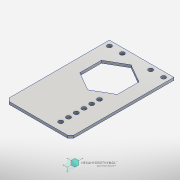
# Autodesk Inventor part: Z-head-topplate
Saved by Autodesk Inventor 2016 (Build 200138000, 138)
## iProperties
Created: 2015-05-16
Part Number: Z-head-topplate
Material: Aluminum 6061
Document SubType Name: Modeling
Designer: as
Mass: 17.1163 g
Surface Area: 72.6872 cm^2
Volume: 6.33935 cm^3
Density: 2.7 g/cm^3
Appearance: Aluminum - Flat
Author: as
Autodesk Inventor part; units mm, degrees
ref_plane "YZ Plane" through (0, 0, 0) normal (1, 0, 0) x (0, 1, 0)
ref_plane "XZ Plane" through (0, 0, 0) normal (0, 1, 0) x (-1, 0, 0)
ref_plane "XY Plane" through (0, 0, 0) normal (0, 0, 1) x (1, 0, 0)
sketch "Sketch1" plane through (0, 0, 0) normal (0, 0, 1) x (1, 0, 0)
  line L0 (0, 0) -> (50, 0)
  line L1 (50, 0) -> (50, -80)
  line L2 (50, -80) -> (0, -80)
  line L3 (0, -80) -> (0, 0)
  dimension "d0" = 50
  dimension "d1" = 80
  constraints: 8 end point, 2 parallel, 1 horizontal, 1 perpendicular
  measures "d0" distance of L1.end L2.end
  measures "d1" distance of L0.end L1.end
extrude "Extrusion1" add sketch "Sketch1" along normal blind 2
sketch "Sketch2" plane through (0, 0, 2) normal (0, 0, 1) x (1, 0, 0)
  point P0 (36, -4)
  point P1 (14, -4)
  point P2 (4, -4)
  point P3 (46, -4)
hole "Hole1" at (36, -4, 2) at (14, -4, 2) at (4, -4, 2) at (46, -4, 2) direction (0, 0, -1) diameter 3.4 depth 2
sketch "Sketch3" plane through (0, 0, 2) normal (0, 0, 1) x (1, 0, 0)
  point P0 (36, -43.66)
hole "Hole3" at (36, -43.66, 2) direction (0, 0, -1) diameter 3.4 depth 2
sketch "Sketch4" plane through (0, 0, 2) normal (0, 0, 1) x (1, 0, 0)
  line L0 (39.5492, -16.6) -> (39.5492, -33.4)
  line L1 (39.5492, -33.4) -> (25, -41.8)
  line L2 (25, -41.8) -> (10.4508, -33.4)
  line L3 (10.4508, -33.4) -> (10.4508, -16.6)
  line L4 (10.4508, -16.6) -> (25, -8.2)
  line L5 (25, -8.2) -> (39.5492, -16.6)
  line L6 (50, -80) -> (50, 0) projected
  line L7 (0, -80) -> (50, -80) projected
  line L8 (50, 0) -> (0, 0) construction
  line L9 (0, 0) -> (0, -80) construction
  point P0 (25, -25)
  dimension "d20" = 16.8
  dimension "d24" = 25
  dimension "d25" = 55
  dimension "d27" = 25
  dimension "d30" = 8.2
  constraints: 12 end point, 1 parallel, 13 other
  measures "d20" distance of L0.start L0.end
  measures "d24" distance from line of L8 point (25, -25)
  measures "d25" distance from line of L7 point (25, -25)
  measures "d27" distance from line of point (25, -25) L9
  measures "d30" distance from line of L8 L4.end
extrude "Extrusion2" cut sketch "Sketch4" against normal blind 10
pattern_linear "Rectangular Pattern4" count 6 spacing 6 along (0, -1, 0) of "Hole3"
chamfer "Chamfer1" distance 2.5 angle 45 2 edges at (50, -80, 1) (0, -80, 1)
body "Solid1"
